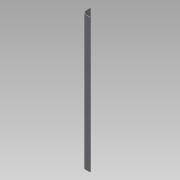
# Autodesk Inventor part: Cart_Side_Beam
Saved by Autodesk Inventor 2015 (Build 190159000, 159)
## iProperties
Created: 2015-05-21
Part Number: Cart_Side_Beam
Material: Generic
Document SubType Name: Modeling
Designer: Joe Sheldon
Density: 1 g/cm^3
Appearance: Default
Author: Joe Sheldon
Autodesk Inventor part; units mm, degrees
ref_plane "YZ Plane" through (0, 0, 0) normal (1, 0, 0) x (0, 1, 0)
ref_plane "XZ Plane" through (0, 0, 0) normal (0, 1, 0) x (-1, 0, 0)
ref_plane "XY Plane" through (0, 0, 0) normal (0, 0, 1) x (1, 0, 0)
sketch "Sketch1" plane through (0, 0, 0) normal (0, 1, 0) x (-1, 0, 0)
  line L0 (0, 0) -> (-38.1, 0)
  line L1 (-38.1, 0) -> (-38.1, -38.1)
  line L2 (-38.1, -38.1) -> (0, -38.1)
  line L3 (0, -38.1) -> (0, 0)
  dimension "d0" = 38.1
  dimension "d1" = 38.1
  constraints: 8 end point, 2 parallel, 1 horizontal, 1 perpendicular
  measures "d0" distance of L2.end L1.end
  measures "d1" distance of L1.end L0.end
extrude "Extrusion1" add sketch "Sketch1" along normal blind 25.4
fillet "Fillet1" radius 19.05 1 edges at (0, 12.7, 0)
sketch "Sketch2" plane through (0, 25.4, 0) normal (0, 1, 0) x (1, 0, 0)
  arc A0 (0, 19.05) -> (19.05, 0) centre (19.05, 19.05) ccw projected
  line L0 (0, 38.1) -> (0, 19.05) projected
  line L1 (38.1, 38.1) -> (0, 38.1) projected
  line L2 (38.1, 0) -> (38.1, 38.1) projected
  line L3 (19.05, 0) -> (38.1, 0) projected
  arc A1 (-2.8591, 19.05) -> (19.05, -2.8591) centre (19.05, 19.05) ccw
  line L4 (-2.8591, 19.05) -> (-2.8591, 40.9591)
  line L5 (-2.8591, 40.9591) -> (40.9591, 40.9591)
  line L6 (40.9591, 40.9591) -> (40.9591, -2.8591)
  line L7 (40.9591, -2.8591) -> (19.05, -2.8591)
  line L8 (0, 38.1) -> (0, 40.9591)
  line L9 (38.1, 0) -> (40.9591, 0)
  point P0 (0, 0)
  constraints: 12 end point, 2 point on circle, 2 point on line, 1 centre point, 1 perpendicular, 1 vertical, 4 other
extrude "Extrusion2" add sketch "Sketch2" along normal blind 44.45 contours A0 L3 L9 L6 L7 A1 L4 L5 L8 L0
sketch "Sketch3" plane through (0, 25.4, 0) normal (0, 1, 0) x (1, 0, 0)
  arc A0 (0, 19.05) -> (19.05, 0) centre (19.05, 19.05) ccw projected
  line L0 (19.05, 0) -> (38.1, 0) projected
  line L1 (38.1, 0) -> (38.1, 38.1) projected
  line L2 (38.1, 38.1) -> (0, 38.1) projected
  line L3 (0, 38.1) -> (0, 19.05) projected
  point P0 (0, 0)
extrude "Extrusion3" cut sketch "Sketch3" against normal blind 44.45
sketch "Sketch4" plane through (0, 69.85, 0) normal (0, 1, 0) x (1, 0, 0)
  arc A0 (0, 19.05) -> (19.05, 0) centre (19.05, 19.05) ccw projected
  line L0 (0, 19.05) -> (0, 40.9591) projected
  line L1 (0, 40.9591) -> (-2.8591, 40.9591) projected
  line L2 (-2.8591, 40.9591) -> (-2.8591, 19.05) projected
  arc A1 (-2.8591, 19.05) -> (19.05, -2.8591) centre (19.05, 19.05) ccw projected
  line L3 (19.05, -2.8591) -> (40.9591, -2.8591) projected
  line L4 (40.9591, -2.8591) -> (40.9591, 0) projected
  line L5 (40.9591, 0) -> (19.05, 0) projected
  point P0 (0, 0)
extrude "Extrusion4" add sketch "Sketch4" along normal blind 660.4
body "Solid1"
